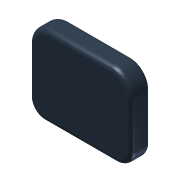
# Autodesk Inventor part: router
Saved by Autodesk Inventor 2012 (Build 160160000, 160)
## iProperties
Created: 2012-05-06
Part Number: router
Material: Default
Document SubType Name: Modeling
Designer: Antonella Wilby
Density: 1 g/cm^3
Author: Antonella Wilby
Autodesk Inventor part; units mm, degrees
ref_plane "YZ Plane" through (0, 0, 0) normal (1, 0, 0) x (0, 1, 0)
ref_plane "XZ Plane" through (0, 0, 0) normal (0, 1, 0) x (-1, 0, 0)
ref_plane "XY Plane" through (0, 0, 0) normal (0, 0, 1) x (1, 0, 0)
sketch "Sketch1" plane through (0, 0, 0) normal (0, 0, 1) x (1, 0, 0)
  line L0 (-6.5727, 23.0598) -> (69.6273, 23.0598)
  line L1 (95.0273, -2.3402) -> (95.0273, -59.4902)
  line L2 (75.9773, -78.5402) -> (-12.9227, -78.5402)
  line L3 (-31.9727, -59.4902) -> (-31.9727, -2.3402)
  arc A0 (-6.5727, 23.0598) -> (-31.9727, -2.3402) centre (-6.5727, -2.3402) ccw
  arc A1 (95.0273, -2.3402) -> (69.6273, 23.0598) centre (69.6273, -2.3402) ccw
  arc A2 (-31.9727, -59.4902) -> (-12.9227, -78.5402) centre (-12.9227, -59.4902) ccw
  arc A3 (75.9773, -78.5402) -> (95.0273, -59.4902) centre (75.9773, -59.4902) ccw
  point P0 (0, 0)
  point P1 (-31.9727, 23.0598)
  point P2 (95.0273, 23.0598)
  point P3 (-31.9727, -78.5402)
  dimension "d0" = 127
  dimension "d1" = 101.6
  dimension "d2" = 25.4
  dimension "d3" = 19.05
  constraints: 8 end point, 8 point on circle, 8 tangent, 6 point on line, 4 centre point, 2 equal radius, 2 parallel, 1 horizontal, 1 perpendicular
  measures "d0" distance of point (-31.973, 23.06) point (95.027, 23.06)
  measures "d1" distance of point (-31.973, -78.54) point (-31.973, 23.06)
  measures "d2" radius of A0
  measures "d3" radius of A2
extrude "Extrusion1" add sketch "Sketch1" along normal blind 25.4
fillet "Fillet1" radius 6.35 16 edges at (-26.3931, -72.9606, 25.4) (-31.9727, -30.9152, 25.4) (-24.5332, 15.6203, 25.4) (31.5273, 23.0598, 25.4) (87.5878, 15.6203, 25.4) (95.0273, -30.9152, 25.4) (89.4477, -72.9606, 25.4) (31.5273, -78.5402, 25.4) (89.4477, -72.9606, 0) (95.0273, -30.9152, 0) (87.5878, 15.6203, 0) (31.5273, 23.0598, 0) (-24.5332, 15.6203, 0) (-31.9727, -30.9152, 0) (-26.3931, -72.9606, 0) (31.5273, -78.5402, 0)
body "Solid1"
